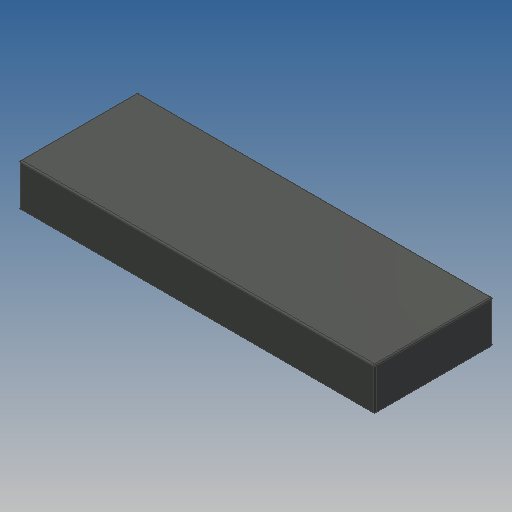
# Autodesk Inventor part: 63864-DkBluishGray
Saved by Autodesk Inventor 2022.2 (Build 262287000, 287)
## iProperties
Created: 2014-06-03
Part Number: 63864-DkBluishGray
Material: ABS Plastic
Document SubType Name: Modeling
Designer: D. Kohfeld
Density: 1.06 g/cm^3
Appearance: DkBluishGray
Mass: 0.471182 g
Surface Area: 6.66198 cm^2
Volume: 0.444511 cm^3
Author: D. Kohfeld
Autodesk Inventor part; units mm, degrees
ref_plane "YZ Plane" through (0, 0, 0) normal (1, 0, 0) x (0, 1, 0)
ref_plane "XZ Plane" through (0, 0, 0) normal (0, 1, 0) x (-1, 0, 0)
ref_plane "XY Plane" through (0, 0, 0) normal (0, 0, 1) x (1, 0, 0)
sketch "Sketch2" plane through (0, 0, 0) normal (0, 1, 0) x (-1, 0, 0)
  line L0 (-12, 4) -> (12, 4)
  line L1 (12, 4) -> (12, -4)
  line L2 (12, -4) -> (-12, -4)
  line L3 (-12, -4) -> (-12, 4)
  point P0 (0, 0)
  point P1 (0, 4)
  point P2 (-12, 0)
  dimension "d0" = 24
  dimension "d1" = 8
  constraints: 8 end point, 2 midpoint, 2 parallel, 1 horizontal, 1 horizontal alignment, 1 perpendicular, 1 vertical alignment
  measures "d0" distance of L1.end L2.end
  measures "d1" distance of L2.end L0.start
extrude "Extrusion1" add sketch "Sketch2" along normal blind 3.2
sketch "Sketch3" plane through (0, 0, 0) normal (0, -1, 0) x (1, 0, 0)
  line L0 (12, 4) -> (-12, 4) projected
  line L1 (-12, 4) -> (-12, -4) projected
  line L2 (-10.4, 2.4) -> (10.4, 2.4)
  line L3 (10.4, 2.4) -> (10.4, -2.4)
  line L4 (10.4, -2.4) -> (-10.4, -2.4)
  line L5 (-10.4, -2.4) -> (-10.4, 2.4)
  circle A0 centre (-4, 4) radius 3.2569
  circle A1 centre (-4, 4) radius 2.4
  line L6 (-12, -4) -> (12, -4) projected
  circle A2 centre (-4, 0) radius 1.6
  line L7 (12, -4) -> (12, 4) projected
  line L8 (-8, 0) -> (0, 0) construction
  line L9 (0, 0) -> (8, 0) construction
  line L10 (-11.6, 3.6) -> (11.6, 3.6)
  line L11 (11.6, 3.6) -> (11.6, -3.6)
  line L12 (11.6, -3.6) -> (-11.6, -3.6)
  line L13 (-11.6, -3.6) -> (-11.6, 3.6)
  point P0 (-10.4, 0)
  point P1 (0, 2.4)
  point P2 (-4, 0)
  point P3 (0, 3.6)
  point P4 (-11.6, 0)
  dimension "d8" = 1.6
  dimension "d60" = 6.5137
  dimension "d61" = 4.8
  dimension "d62" = 1.6
  dimension "d75" = 8
  dimension "d76" = 8
  dimension "d86" = 3.2
  dimension "d89" = 8
  dimension "d95" = 0.4
  dimension "d96" = 0.4
  constraints: 20 end point, 5 coincident, 5 midpoint, 5 parallel, 3 centre point, 3 perpendicular, 2 collinear, 2 horizontal, 2 horizontal alignment, 2 vertical alignment
  measures "d8" distance between parallel lines of L1 L5
  measures "d60" diameter of A0
  measures "d61" diameter of A1
  measures "d62" distance between parallel lines of L0 L2
  measures "d75" distance from line of A0.centre L1
  measures "d76" distance from line of A0.centre L6
  measures "d86" diameter of A2
  measures "d89" distance of L8.start L8.end
  measures "d95" distance between parallel lines of L0 L10
  measures "d96" distance between parallel lines of L1 L13
extrude "Extrusion2" cut sketch "Sketch3" against normal blind 1.6 contours A0 A2 A1 L2 | L2 L3 L4 L5 A0 A2 | A1 L2 | L2 A1 A2 A0 | A2 A0 | A0 A2
extrude "Extrusion7" cut sketch "Sketch3" against normal blind 0.4 contours L7 L6 L1 L0 A0 L10 L13 L12 L11 | A0 L10 A1 L0 | A1 L10 L0 | L0 A1 L10 A0
fillet "Fillet1" radius 0.1 8 edges at (-12, 1.8, 4) (0, 3.2, 4) (-12, 3.2, 0) (0, 3.2, -4) (12, 3.2, 0) (12, 1.8, 4) (12, 1.8, -4) (-12, 1.8, -4)
equation "\"d4\" = 0.333333 * lh"
equation "\"d8\" = d62"
equation "\"d60\" = tubeod"
equation "\"d61\" = kd"
equation "\"d62\" = wall"
equation "\"d75\" = lu"
equation "\"d76\" = d75"
equation "\"d86\" = pd"
equation "\"d89\" = lu"
equation "\"d95\" = gw"
equation "\"d96\" = gw"
equation "\"d11\" = 0.333333 * lh - topthk"
equation "\"d97\" = gh"
equation "\"lh\" = 9.6"
equation "\"tubeod\" = 6.513708"
equation "\"kd\" = 4.8"
equation "\"wall\" = 1.6"
equation "\"lu\" = 8"
equation "\"pd\" = 3.2"
equation "\"gw\" = 0.4"
equation "\"topthk\" = 1.6"
equation "\"gh\" = 0.4"
body "Solid1"
